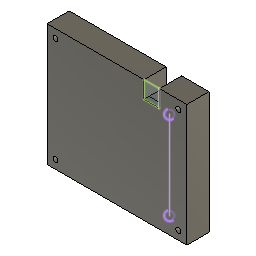
back_01 (Autodesk Fusion 360 design; units mm, degrees)
part number: 2026-02-06-21-37-17-528
Autodesk Fusion 360 part; units mm, degrees
sketch "Sketch3" plane through (0, 0, 0) normal (0, 1, 0) x (1, 0, 0)
sketch "Sketch4" plane through (0, 0, 0) normal (0, 1, 0) x (1, 0, 0)
sketch "Sketch5" plane through (0, 0, 0) normal (0, 1, 0) x (1, 0, 0)
sketch "Sketch6" plane through (0, 0, 0) normal (0, 1, 0) x (1, 0, 0)
  line L0 (-42.6895, -21.6471) -> (19.3705, -21.6471)
  line L1 (19.3705, -21.6471) -> (19.3705, 29.8529)
  line L2 (19.3705, 29.8529) -> (-42.6895, 29.8529)
  line L3 (-42.6895, 29.8529) -> (-42.6895, -21.6471)
  line L4 (-52.6895, -31.6471) -> (29.3705, -31.6471)
  line L5 (29.3705, -31.6471) -> (29.3705, 39.8529)
  line L6 (29.3705, 39.8529) -> (-52.6895, 39.8529)
  line L7 (-52.6895, 39.8529) -> (-52.6895, -31.6471)
  circle A0 centre (-47.6895, -26.6471) radius 1.45
  circle A1 centre (24.3705, -26.6471) radius 1.45
  circle A2 centre (-47.6895, 34.8529) radius 1.45
  circle A3 centre (24.3705, 34.8529) radius 1.45
  dimension "d52" = 51.5
  dimension "d53" = 62.06
  dimension "d54" = 10
  dimension "d55" = 10
  dimension "d56" = 10
  dimension "d57" = 10
  dimension "d58" = 2.9
  dimension "d59" = 5
  dimension "d60" = 5
  dimension "d61" = 2.9
  dimension "d62" = 5
  dimension "d63" = 5
  dimension "d64" = 2.9
  dimension "d65" = 5
  dimension "d66" = 5
  dimension "d67" = 2.9
  dimension "d68" = 5
  dimension "d69" = 5
  constraint horizontal L0
  constraint vertical L1
  constraint horizontal L2
  constraint vertical L3
  constraint horizontal L4
  constraint vertical L5
  constraint horizontal L6
  constraint vertical L7
  measures "d52" distance of L0.start L2.end
  measures "d53" distance of L1 L3
  measures "d54" distance of L0 L4
  measures "d55" distance of L1 L5
  measures "d56" distance of L3 L7
  measures "d57" distance of L2 L6
  measures "d58" diameter of A0
  measures "d59" distance of L4 A0.centre
  measures "d60" distance of L7 A0.centre
  measures "d61" diameter of A1
  measures "d62" distance of L5 A1.centre
  measures "d63" distance of L4 A1.centre
  measures "d64" diameter of A2
  measures "d65" distance of L6 A2.centre
  measures "d66" distance of L7 A2.centre
  measures "d67" diameter of A3
  measures "d68" distance of L5 A3.centre
  measures "d69" distance of L6 A3.centre
extrude "Extrude6" add sketch "Sketch6" along normal blind 13
extrude "Extrude7" add sketch "Sketch6" along normal blind 3 contours L0 L1 L2 L3
sketch "Sketch7" plane through (0, 0, 0) normal (0, 1, 0) x (1, 0, 0)
  line L0 (13.2505, -31.6778) -> (4.2505, -31.6778)
  line L1 (4.2505, -31.6778) -> (4.2505, -21.6778)
  line L2 (4.2505, -21.6778) -> (13.2505, -21.6778)
  line L3 (13.2505, -21.6778) -> (13.2505, -31.6778)
  line L4 (19.3705, -21.6471) -> (19.3705, 29.8529)
  dimension "d74" = 10
  dimension "d75" = 6.12
  dimension "d76" = 9
  constraint horizontal L0
  constraint vertical L1
  constraint horizontal L2
  constraint vertical L3
  measures "d74" distance of L0.start L2.end
  measures "d75" distance of L3 L4
  measures "d76" distance of L1 L3
sketch "Sketch8" plane through (0, 0, 0) normal (0, 1, 0) x (1, 0, 0)
sketch "eee" plane through (0, 0, 0) normal (0, 1, 0) x (1, 0, 0)
  line L0 (13.3073, -31.6778) -> (4.2109, -31.6778)
  line L1 (4.2109, -31.6778) -> (4.2109, -21.6873)
  line L2 (4.2109, -21.6873) -> (13.3073, -21.6873)
  line L3 (13.3073, -21.6873) -> (13.3073, -31.6778)
  line L4 (4.2505, -21.6778) -> (13.2505, -21.6778)
  dimension "d77" = 10
  constraint horizontal L0
  constraint vertical L1
  constraint horizontal L2
  constraint vertical L3
  measures "d77" distance of L0 L4
extrude "Extrude8" cut sketch "eee" along normal blind 13
